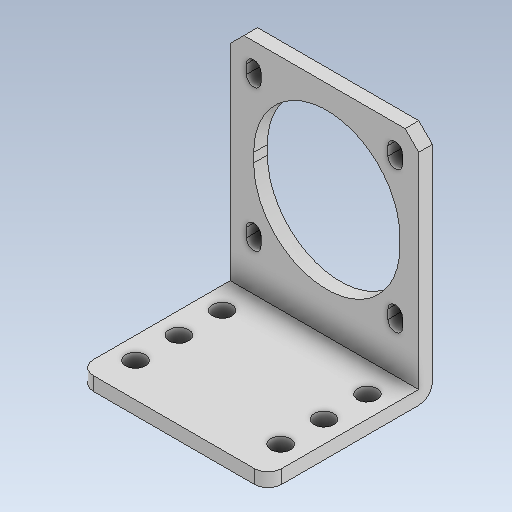
# Autodesk Inventor part: ブラケット
Saved by Autodesk Inventor 2020 (Build 240168000, 168)
## iProperties
Created: 2020-06-21
Part Number: ブラケット
Material: 一般
Document SubType Name: Modeling
Designer: bsat3
Density: 1 g/cm^3
Appearance: 既定
Author: bsat3
Autodesk Inventor part; units mm, degrees
ref_plane "YZ Plane" through (0, 0, 0) normal (1, 0, 0) x (0, 1, 0)
ref_plane "XZ Plane" through (0, 0, 0) normal (0, 1, 0) x (-1, 0, 0)
ref_plane "XY Plane" through (0, 0, 0) normal (0, 0, 1) x (1, 0, 0)
sketch "スケッチ1" plane through (0, 0, 0) normal (0, 0, 1) x (1, 0, 0)
  line L0 (20.15, -28.9) -> (-21.15, -28.9)
  line L1 (-21.15, -28.9) -> (-21.15, 22.1)
  line L2 (-21.15, 22.1) -> (20.15, 22.1)
  line L3 (20.15, 22.1) -> (20.15, -28.9)
  line L4 (-16, -1) -> (-16, 1)
  line L5 (16, 1) -> (16, -1)
  line L6 (16, -1) -> (-16, 1) construction
  line L7 (-16, -1) -> (16, 1) construction
  arc A0 (-16, -1) -> (16, -1) centre (0, -1) ccw
  arc A1 (16, 1) -> (-16, 1) centre (0, 1) ccw
  line L8 (-16, 1) -> (-15.8745, 1)
  line L9 (15.8745, 1) -> (16, 1)
  line L10 (16, -1) -> (15.8745, -1)
  line L11 (-15.8745, -1) -> (-16, -1)
  arc A2 (-14.4, 17) -> (-17.6, 17) centre (-16, 17) ccw
  line L12 (-14.4, 17) -> (-14.4, 15)
  line L13 (-17.6, 15) -> (-17.6, 17)
  arc A3 (-17.6, 15) -> (-14.4, 15) centre (-16, 15) ccw
  arc A4 (16.6, 17) -> (13.4, 17) centre (15, 17) ccw
  line L14 (13.4, 15) -> (13.4, 17)
  arc A5 (13.4, 15) -> (16.6, 15) centre (15, 15) ccw
  line L15 (16.6, 17) -> (16.6, 15)
  arc A6 (-14.4, -14) -> (-17.6, -14) centre (-16, -14) ccw
  line L16 (-17.6, -16) -> (-17.6, -14)
  arc A7 (-17.6, -16) -> (-14.4, -16) centre (-16, -16) ccw
  line L17 (-14.4, -14) -> (-14.4, -16)
  arc A8 (16.6, -14) -> (13.4, -14) centre (15, -14) ccw
  line L18 (13.4, -16) -> (13.4, -14)
  arc A9 (13.4, -16) -> (16.6, -16) centre (15, -16) ccw
  line L19 (16.6, -14) -> (16.6, -16)
  point P0 (0, 0)
  point P1 (13.4, -15)
  point P2 (16.6, -15)
  dimension "d5" = 41.3
  dimension "d6" = 51
  dimension "d7" = 2
  dimension "d9" = 16
  dimension "d12" = 2
  dimension "d13" = 1.6
  dimension "d14" = 1.6
  dimension "d17" = 31
  dimension "d20" = 31
  dimension "d29" = 5.15
  dimension "d30" = 14.9
  constraints: 40 end point, 24 point on circle, 10 centre point, 8 parallel, 4 horizontal, 4 midpoint, 3 perpendicular, 1 vertical, 33 other
  measures "d5" distance of L1.end L2.end
  measures "d6" distance of L0.end L1.end
  measures "d7" distance of L5.start L5.end
  measures "d9" radius of A1
  measures "d12" distance of L12.start L12.end
  measures "d13" radius of A2
  measures "d14" radius of A3
  measures "d17" distance of A2.centre A4.centre
  measures "d20" distance of A2.centre A6.centre
  measures "d29" distance from line of L3 A9.centre
  measures "d30" distance from line of L0 A8.centre
extrude "押し出し1" add sketch "スケッチ1" along normal blind 3
sketch "スケッチ2" plane through (0, 0, 3) normal (0, 0, 1) x (1, 0, 0)
  line L0 (-21.15, -28.9) -> (20.15, -28.9) projected
  line L1 (-21.15, -28.9) -> (20.15, -28.9)
  line L2 (20.15, -28.9) -> (20.15, -25.9)
  line L3 (20.15, -25.9) -> (-21.15, -25.9)
  line L4 (-21.15, -25.9) -> (-21.15, -28.9)
  point P0 (0, 0)
  dimension "d25" = 3
  constraints: 8 end point, 2 parallel, 1 horizontal, 1 perpendicular
  measures "d25" distance of L1.end L2.end
extrude "押し出し2" add sketch "スケッチ2" along normal blind 33
sketch "スケッチ3" plane through (-21.15, -28.9, 0) normal (0, -1, 0) x (1, 0, 0)
  line L0 (4.75, 19) -> (36.55, 19)
  line L1 (36.55, 19) -> (36.55, 9.5)
  line L2 (36.55, 9.5) -> (4.75, 9.5)
  line L3 (4.75, 9.5) -> (4.75, 19)
  line L4 (0, 0) -> (41.3, 0) projected
  line L5 (41.3, 0) -> (41.3, 36) projected
  point P0 (21.15, 0)
  point P1 (36.55, 28.5)
  point P2 (4.75, 28.5)
  dimension "d31" = 9.5
  dimension "d32" = 9.5
  dimension "d33" = 31.8
  dimension "d34" = 4.75
  dimension "d42" = 28.5
  constraints: 8 end point, 4 coincident, 2 parallel, 2 point on line, 1 horizontal, 1 horizontal alignment, 1 perpendicular
  measures "d31" distance between parallel lines of L4 L2
  measures "d32" distance of L2.end L0.start
  measures "d33" distance of L0.start L0.end
  measures "d34" distance between parallel lines of L5 L1
  measures "d42" distance from line of point (36.55, 28.5) L4
hole "穴1" at (-16.4, -28.9, 9.5) at (-16.4, -28.9, 19) at (15.4, -28.9, 9.5) at (15.4, -28.9, 19) at (15.4, -28.9, 28.5) at (-16.4, -28.9, 28.5) direction (0, 1, 0) diameter 4.3 end through all
chamfer "面取り1" distance 3 angle 45 2 edges at (20.15, 22.1, 1.5) (-21.15, 22.1, 1.5)
fillet "フィレット1" radius 3 3 edges at (-21.15, -27.4, 36) (20.15, -27.4, 36) (-0.5, -28.9, 0)
